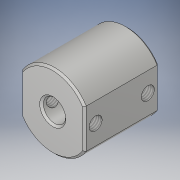
# Autodesk Inventor part: КВ33.000.106 - Муфта
Saved by Autodesk Inventor 2019 (Build 230136000, 136)
## iProperties
Created: 2021-03-22
Part Number: КВ33.000.106 - Муфта
Material: Aluminum 6061
Document SubType Name: Modeling
Designer: Петров Иван
Density: 2.7 g/cm^3
Appearance: Aluminum - Flat
Mass: 13.9072 g
Surface Area: 22.5864 cm^2
Volume: 5.15082 cm^3
Author: Петров Иван
Autodesk Inventor part; units mm, degrees
ref_plane "YZ Plane" through (0, 0, 0) normal (1, 0, 0) x (0, 1, 0)
ref_plane "XZ Plane" through (0, 0, 0) normal (0, 1, 0) x (-1, 0, 0)
ref_plane "XY Plane" through (0, 0, 0) normal (0, 0, 1) x (1, 0, 0)
sketch "Sketch1" plane through (0, 0, 0) normal (0, 0, 1) x (1, 0, 0)
  circle A0 centre (0, 0) radius 10
  dimension "d0" = 20
  constraints: 1 centre point, 1 coincident
  measures "d0" diameter of A0
extrude "Extrusion1" add sketch "Sketch1" along normal blind 20
sketch "Sketch2" plane through (0, 0, 20) normal (0, 0, 1) x (1, 0, 0)
  circle A0 centre (0, 0) radius 3
  dimension "d3" = 6
  constraints: 1 centre point, 1 coincident
  measures "d3" diameter of A0
extrude "Extrusion2" cut sketch "Sketch2" against normal blind 7.5
sketch "Sketch3" plane through (0, 0, 0) normal (0, 0, -1) x (-1, 0, 0)
  circle A0 centre (0, 0) radius 3 projected
  circle A1 centre (0, 0) radius 2.5
  dimension "d6" = 5
  constraints: 1 centre point, 1 coincident
  measures "d6" diameter of A1
extrude "Extrusion3" cut sketch "Sketch3" against normal through all contours A1
sketch "Sketch4" plane through (0, 0, 0) normal (1, 0, 0) x (0, 1, 0)
  circle A0 centre (0, 3) radius 1.5
  line L0 (-10, 0) -> (10, 0) projected
  circle A1 centre (0, 17) radius 1.5
  line L1 (10, 20) -> (-10, 20) projected
  point P0 (0, 0)
  dimension "d9" = 3
  dimension "d10" = 3
  dimension "d11" = 3
  dimension "d12" = 3
  constraints: 2 centre point
  measures "d9" diameter of A0
  measures "d10" distance from line of L0 A0.centre
  measures "d11" diameter of A1
  measures "d12" distance from line of L1 A1.centre
sketch "Sketch5" plane through (0, 0, 20) normal (0, 0, 1) x (1, 0, 0)
  circle A0 centre (0, 0) radius 10 projected
  line L0 (-8.5, -5.2678) -> (-8.5, 5.2678)
  dimension "d48" = 8.5
  constraints: 2 end point, 2 point on circle, 1 vertical
  measures "d48" distance from line of point (0, 0) L0
extrude "Extrusion5" cut sketch "Sketch5" against normal blind 21.25 contours L0 A0 picked at (-8.817, 1.0892)
mirror "Mirror1" about plane through (0, 0, 0) normal (1, 0, 0) of "Extrusion5"
chamfer "Chamfer1" distance 0.5 angle 45 2 edges at (-3, 0, 20) (2.5, 0, 0)
chamfer "Chamfer2" distance 0.5 angle 45 8 edges at (0, 10, 20) (8.5, 0, 20) (0, 10, 0) (8.5, 0, 0) (0, -10, 0) (-8.5, 0, 0) (-8.5, 0, 20) (0, -10, 20)
hole "Hole1" at (0, 0, 17) at (0, 0, 3) direction (-1, 0, 0) diameter 3.5 end through all both
thread "Thread5" size "M3.5x0.6" class "6H" standard "ANSI Metric M Profile" full length
thread "Thread6" size "M3.5x0.6" class "6H" standard "ANSI Metric M Profile" full length
thread "Thread7" size "M3.5x0.6" class "6H" standard "ANSI Metric M Profile" full length
thread "Thread8" size "M3.5x0.6" class "6H" standard "ANSI Metric M Profile" full length
body "Solid1"
